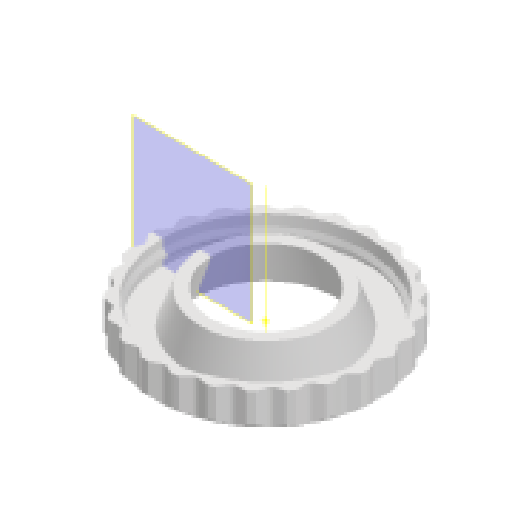
# Autodesk Inventor part: 20_Cube_4_insert_polfilter_nut
Saved by Autodesk Inventor 2025.1 (Build 291241000, 241)
## iProperties
Created: 2024-10-07
Part Number: 20_Cube_4_insert_polfilter_nut
Material: Generic
Document SubType Name: Modeling
Designer: diederichbenedict
Density: 1 g/cm^3
Appearance: Default
Author: diederichbenedict
Autodesk Inventor part; units mm, degrees
ref_plane "YZ Plane" through (0, 0, 0) normal (1, 0, 0) x (0, 1, 0)
ref_plane "XY Plane" through (0, 0, 0) normal (0, 0, 1) x (1, 0, 0)
ref_plane "Work Plane2" through (13.3532, -14.5473, -9.2) normal (0, 1, 0) x (-1, 0, 0)
sketch "Sketch1" plane through (13.3532, -14.5473, -9.2) normal (0, 1, 0) x (-1, 0, 0)
  line L0 (-18.7, 5) -> (-18.7, 1) construction
  line L1 (-17.9929, 2.2929) -> (-17.9929, 2.7929)
  line L2 (-18.7, 1) -> (-17.7, 0)
  line L3 (-17.9929, 2.2929) -> (-18.7, 1.5858)
  line L4 (-17.7707, -0.0707) -> (-18.8, 0.9586)
  line L5 (-18.8, 0.9586) -> (-18.8, 5)
  line L6 (-18.7707, 1.6565) -> (-18.0929, 2.3343)
  line L7 (-18.0929, 2.3343) -> (-18.0929, 2.7929)
  line L8 (-18.0929, 2.7929) -> (-18.8, 3.5)
  line L9 (-18.8, 3.5) -> (-18.8, 1.6272)
  line L10 (-18.0929, 2.3343) -> (-18.8, 1.6272)
  point P0 (13.3532, 9.2)
  dimension "d0" = 0.1
  dimension "d1" = 0.1
  constraints: 22 end point, 3 point on line, 2 vertical, 1 parallel, 8 other
  measures "d0" distance between parallel lines of L2 L4
  measures "d1" distance between parallel lines of L3 L6
coil "Coil1" sketch "Sketch1" operation add axis through (13.3532, -14.5473, -8.2) along (0, 0, -1) pitch 3 turns 1.5 hand right
sketch "Sketch2" plane through (0, -14.5473, 0) normal (0, 1, 0) x (-1, 0, 0)
  line L0 (5.4468, -7.2) -> (5.4468, -12.0728) projected
  line L1 (-32.1532, -5.7) -> (-32.1532, -7.5728) projected
  line L2 (-32.1532, -5.7) -> (-32.1532, -10.5728) projected
  line L3 (-32.1532, -5.7) -> (-34.1532, -5.7)
  line L4 (-34.1532, -5.7) -> (-34.1532, -11.0728)
  line L5 (-33.1532, -12.0728) -> (-32.1532, -12.0728)
  line L6 (-32.1532, -12.0728) -> (-32.1532, -5.7)
  line L7 (-34.1532, -12.0728) -> (-26.1532, -12.0728)
  line L8 (-26.1532, -12.0728) -> (-26.1532, -10.0728)
  line L9 (-26.1532, -10.0728) -> (-34.1532, -10.0728)
  line L10 (-34.1532, -10.0728) -> (-34.1532, -12.0728)
  line L11 (-13.3532, -14.4874) -> (-13.3532, 2.4146) projected
  line L12 (-33.1532, -12.0728) -> (-34.1532, -11.0728)
  line L13 (-22.3532, 0) -> (-22.3532, -3.9) projected
  line L14 (-26.1532, -12.0728) -> (-23.2414, -4.0728)
  line L15 (-26.1532, -12.0728) -> (-17.6397, -12.0728) construction
  line L16 (-23.2414, -4.0728) -> (-25.3698, -4.0728)
  line L17 (-25.3698, -4.0728) -> (-27.5536, -10.0728)
  line L18 (-32.1532, -5.7) -> (-33.1532, -5.1706)
  line L19 (-33.1532, -5.1706) -> (-34.1532, -5.7)
  point P0 (0, 0)
  point P1 (-32.1532, -10.0728)
  point P2 (-32.6532, -12.0728)
  dimension "d10" = 2
  dimension "d11" = 8
  dimension "d12" = 2
  dimension "d14" = 1
  dimension "d15" = 1
  dimension "d16" = 70
  dimension "d17" = 0
  dimension "d18" = 2
  dimension "d28" = 8
  constraints: 30 end point, 6 parallel, 3 horizontal, 3 point on line, 2 perpendicular, 1 equal length, 1 midpoint
  measures "d10" distance between parallel lines of L4 L6
  measures "d11" distance of L9.end L8.end
  measures "d12" distance of L8.end L7.end
  measures "d14" distance of L5.start L7.start
  measures "d15" distance of L4.end L7.start
  measures "d16" angle of L15 L14
  measures "d17" vertical distance of L0.end point (-32.653, -12.073)
  measures "d18" distance between parallel lines of L17 L14
  measures "d28" distance between parallel lines of L7 L16
revolve "Revolution1" add sketch "Sketch2" angle 360 about axis through (13.3532, -14.5473, -8.2) along (0, 0, 1) contours L1 L2 L9 L4 L3 | L3 L19 L18 | L9 L8 L7 L6 L2 | L2 L6 L5 L12 L4 L9 | L17 L16 L14 L8 L9
sketch "Sketch3" plane through (13.3532, -14.5473, -12.0728) normal (0, 0, -1) x (-1, 0, 0)
  circle A0 centre (0, 0) radius 20.8 projected
  circle A1 centre (-20.8, 0) radius 1
  point P0 (13.3532, 14.5473)
  dimension "d19" = 2
  constraints: 1 centre point, 1 horizontal alignment, 1 other
  measures "d19" diameter of A1
extrude "Extrusion1" cut sketch "Sketch3" against normal through all contours A1 A0 | A0 A1 picked at (-20.4649, 0) picked at (-21.129, 0.0408)
chamfer "Chamfer1" distance 1 angle 45 2 edges at (34.1291, -13.5476, -8.3864) (34.1291, -15.547, -8.3864)
pattern_circular "Circular Pattern1" count 25 over 360 about axis through (13.3532, -14.5473, -8.3864) along (0, 0, 1) of "Extrusion1", "Chamfer1"
ref_plane "Work Plane1" through (-2.3468, -14.5473, -9.2) normal (0, 0, -1) x (-1, 0, 0)
equation "\"d15\" = d14"
body "Solid1"
